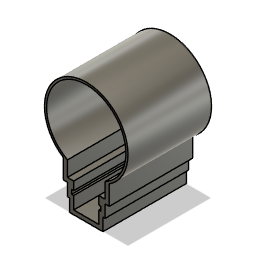
神秘PCB扣具 (Autodesk Fusion 360 design; units mm, degrees)
Autodesk Fusion 360 part; units mm, degrees
sketch "草图1" plane through (0, 0, 0) normal (0, 1, 0) x (1, 0, 0)
  circle A0 centre (0, 0) radius 10
  dimension "d1" = 20
  constraint coincident A0.centre origin
  measures "d1" diameter of A0
extrude "拉伸1" add sketch "草图1" along normal blind 20 makes body 1
sketch "草图2" plane through (0, 20, 0) normal (0, 1, 0) x (-1, 0, 0)
  circle A0 centre (0, 0) radius 10
  circle A1 centre (0, 0) radius 9.5
  dimension "d4" = 19
  constraint concentric A0 A1
  measures "d4" diameter of A1
extrude "拉伸2" cut sketch "草图2" against normal blind 20 contours A1 bodies 1
sketch "草图3" plane through (0, 20, 0) normal (0, 1, 0) x (-1, 0, 0)
  circle A0 centre (0, 0) radius 9.5
  circle A1 centre (0, 0) radius 10
  line L0 (4, 9) -> (-4, 9)
  line L1 (-4, 9) -> (-4, 19)
  line L2 (-4, 19) -> (4, 19)
  line L3 (4, 19) -> (4, 9)
  line L4 (3, 10) -> (-3, 10)
  line L5 (-3, 10) -> (-3, 18)
  line L6 (-3, 18) -> (3, 18)
  line L7 (3, 18) -> (3, 10)
  line L8 (3, 14) -> (3.5, 14)
  line L9 (3.5, 14) -> (3.5, 15)
  line L10 (3.5, 15) -> (3, 15)
  line L11 (3, 15) -> (3, 14)
  line L12 (-3, 14) -> (-3.5, 14)
  line L13 (-3.5, 14) -> (-3.5, 15)
  line L14 (-3.5, 15) -> (-3, 15)
  line L15 (-3, 15) -> (-3, 14)
  dimension "d7" = 8
  dimension "d8" = 4
  dimension "d9" = 9
  dimension "d10" = 10
  dimension "d11" = 1
  dimension "d12" = 1
  dimension "d13" = 1
  dimension "d14" = 1
  dimension "d15" = 0.5
  dimension "d16" = 1
  dimension "d17" = 0.5
  dimension "d18" = 1
  constraint horizontal L0
  constraint vertical L1
  constraint horizontal L2
  constraint vertical L3
  constraint horizontal L4
  constraint vertical L5
  constraint horizontal L6
  constraint vertical L7
  constraint horizontal L8
  constraint vertical L9
  constraint horizontal L10
  constraint vertical L11
  constraint midpoint L7 L8.start
  constraint horizontal L12
  constraint vertical L13
  constraint horizontal L14
  constraint vertical L15
  constraint midpoint L5 L12.start
  measures "d7" distance of L0.start L0.end
  measures "d8" distance of A0.centre L3
  measures "d9" distance of A0.centre L0
  measures "d10" distance of L0 L2
  measures "d11" distance of L0 L4
  measures "d12" distance of L2 L6
  measures "d13" distance of L1 L5
  measures "d14" distance of L3 L7
  measures "d15" distance of L9.end L10.end
  measures "d16" distance of L8 L10
  measures "d17" distance of L13.end L14.end
  measures "d18" distance of L12 L14
extrude "拉伸3" add sketch "草图3" against normal blind 20 contours A1 L1 L2 L3 bodies 1
sketch "草图4" plane through (0, 20, 0) normal (0, 1, 0) x (-1, 0, 0)
  line L0 (-3, 18) -> (3, 18)
  line L1 (3, 14) -> (3, 10)
  line L2 (3, 10) -> (-3, 10)
  line L3 (-3, 10) -> (-3, 14)
  line L4 (4, 9.1652) -> (4, 19)
  line L5 (4, 19) -> (-4, 19)
  line L6 (-4, 19) -> (-4, 9.1652)
  arc A0 (-4, 9.1652) -> (4, 9.1652) centre (0, 0) ccw
  line L7 (3, 14) -> (-3, 14)
  line L8 (-3, 14) -> (-3, 7.5)
  line L9 (-3, 7.5) -> (3, 7.5)
  line L10 (3, 7.5) -> (3, 14)
  line L11 (-3, 14) -> (-3.5, 14)
  line L12 (-3.5, 14) -> (-3.5, 15)
  line L13 (-3.5, 15) -> (-3, 15)
  line L14 (-3, 15) -> (-3, 18)
  line L15 (3, 18) -> (3, 15)
  line L16 (3, 15) -> (3.5, 15)
  line L17 (3.5, 15) -> (3.5, 14)
  line L18 (3.5, 14) -> (3, 14)
  circle A1 centre (0, 0) radius 9.5
  constraint horizontal L7
  constraint vertical L8
  constraint horizontal L9
  constraint vertical L10
  constraint coincident L1.start L7.start
extrude "拉伸4" cut sketch "草图4" against normal blind 20 contours L8 L9 L10 A1 picked at (-0.1243, 1.8358) bodies 1
sketch "草图5" plane through (0, 20, 0) normal (0, 1, 0) x (-1, 0, 0)
  line L0 (3, 10) -> (-3, 10)
  line L1 (-3, 10) -> (-3, 14)
  line L2 (-3, 14) -> (-3.5, 14)
  line L3 (-3.5, 14) -> (-3.5, 15)
  line L4 (-3.5, 15) -> (-3, 15)
  line L5 (-3, 15) -> (-3, 18)
  line L6 (-3, 18) -> (3, 18)
  line L7 (3, 18) -> (3, 15)
  line L8 (3, 15) -> (3.5, 15)
  line L9 (3.5, 15) -> (3.5, 14)
  line L10 (3.5, 14) -> (3, 14)
  line L11 (3, 14) -> (3, 10)
  circle A0 centre (0, 0) radius 9.5
  line L12 (4, 9.1652) -> (4, 19)
  line L13 (4, 19) -> (-4, 19)
  line L14 (-4, 19) -> (-4, 9.1652)
  arc A1 (-4, 9.1652) -> (4, 9.1652) centre (0, 0) ccw
  line L15 (4, 10) -> (-4, 10)
  line L16 (-4, 10) -> (-4, 13)
  line L17 (-4, 13) -> (4, 13)
  line L18 (4, 13) -> (4, 10)
  constraint horizontal L15
  constraint vertical L16
  constraint horizontal L17
  constraint vertical L18
  constraint coincident L14 L16.end
  constraint coincident L12 L15.start
extrude "拉伸5" cut sketch "草图5" against normal blind 20 contours L0 L1 L11 L15 L17 | L11 L12 L15 L17 L18 | L1 L14 L15 L16 L17 bodies 1 makes body 2 at (1.3333, 13.3333, 19)
sketch "草图6" plane through (0, 20, 0) normal (0, 1, 0) x (-1, 0, 0)
  circle A0 centre (0, 0) radius 9.5
  line L0 (4, 10) -> (-4, 10)
  line L1 (-4, 10) -> (-4, 9.1652)
  arc A1 (-4, 9.1652) -> (4, 9.1652) centre (0, 0) ccw
  line L2 (4, 9.1652) -> (4, 10)
  line L3 (5.5, 8) -> (-5.5, 8)
  line L4 (-5.5, 8) -> (-5.5, 13)
  line L5 (-5.5, 13) -> (5.5, 13)
  line L6 (5.5, 13) -> (5.5, 8)
  dimension "d25" = 5
  constraint horizontal L3
  constraint vertical L4
  constraint horizontal L5
  constraint vertical L6
  measures "d25" distance of L3.start L5.end
extrude "拉伸6" add sketch "草图6" against normal blind 20 contours L0 L1 A1 L2 L4 L5 L6 bodies 1 2
sketch "草图7" plane through (0, 20, 0) normal (0, 1, 0) x (-1, 0, 0)
  line L0 (-3, 13) -> (-3, 14)
  line L1 (-3, 14) -> (-3.5, 14)
  line L2 (-3.5, 14) -> (-3.5, 15)
  line L3 (-3.5, 15) -> (-3, 15)
  line L4 (-3, 15) -> (-3, 18)
  line L5 (-3, 18) -> (3, 18)
  line L6 (3, 18) -> (3, 15)
  line L7 (3, 15) -> (3.5, 15)
  line L8 (3.5, 15) -> (3.5, 14)
  line L9 (3.5, 14) -> (3, 14)
  line L10 (3, 14) -> (3, 13)
  line L11 (3, 13) -> (-3, 13)
  circle A0 centre (0, 0) radius 9.5
  line L12 (5.5, 8.3516) -> (5.5, 13)
  line L13 (5.5, 13) -> (4, 13)
  line L14 (4, 13) -> (4, 19)
  line L15 (4, 19) -> (-4, 19)
  line L16 (-4, 19) -> (-4, 13)
  line L17 (-4, 13) -> (-5.5, 13)
  line L18 (-5.5, 13) -> (-5.5, 8.3516)
  arc A1 (-5.5, 8.3516) -> (5.5, 8.3516) centre (0, 0) ccw
  line L19 (4.5, 8.0706) -> (-4.5, 8.0706)
  line L20 (-4.5, 8.0706) -> (-4.5, 12)
  line L21 (-4.5, 12) -> (4.5, 12)
  line L22 (4.5, 12) -> (4.5, 8.0706)
  dimension "d28" = 1
  dimension "d29" = 1
  dimension "d30" = 1
  constraint horizontal L19
  constraint vertical L20
  constraint horizontal L21
  constraint vertical L22
  measures "d28" distance of L12 L22
  measures "d29" distance of L18 L20
  measures "d30" distance of L13 L21
extrude "拉伸7" cut sketch "草图7" against normal blind 20 contours A0 L20 L21 L22 bodies 1
sketch "草图8" plane through (0, 20, 0) normal (0, 1, 0) x (-1, 0, 0)
  line L0 (4.5, 12) -> (4.5, 8.3666)
  arc A0 (-4.5, 8.3666) -> (4.5, 8.3666) centre (0, 0) ccw
  line L1 (-4.5, 8.3666) -> (-4.5, 12)
  line L2 (-4.5, 12) -> (4.5, 12)
  line L3 (-3, 13) -> (-3, 14)
  line L4 (-3, 14) -> (-3.5, 14)
  line L5 (-3.5, 14) -> (-3.5, 15)
  line L6 (-3.5, 15) -> (-3, 15)
  line L7 (-3, 15) -> (-3, 18)
  line L8 (-3, 18) -> (3, 18)
  line L9 (3, 18) -> (3, 15)
  line L10 (3, 15) -> (3.5, 15)
  line L11 (3.5, 15) -> (3.5, 14)
  line L12 (3.5, 14) -> (3, 14)
  line L13 (3, 14) -> (3, 13)
  line L14 (3, 13) -> (-3, 13)
  line L15 (5.5, 8.3516) -> (5.5, 13)
  line L16 (5.5, 13) -> (4, 13)
  line L17 (4, 13) -> (4, 19)
  line L18 (4, 19) -> (-4, 19)
  line L19 (-4, 19) -> (-4, 13)
  line L20 (-4, 13) -> (-5.5, 13)
  line L21 (-5.5, 13) -> (-5.5, 8.3516)
  arc A1 (-5.5, 8.3516) -> (5.5, 8.3516) centre (0, 0) ccw
  line L22 (3, 12) -> (-3, 12)
  line L23 (-3, 12) -> (-3, 13)
  line L24 (-3, 13) -> (3, 13)
  line L25 (3, 13) -> (3, 12)
  constraint horizontal L22
  constraint vertical L23
  constraint horizontal L24
  constraint vertical L25
  constraint coincident L3.start L14.end
  constraint coincident L2 L22.start
extrude "拉伸8" cut sketch "草图8" against normal blind 20 contours L2 L14 L22 L23 L24 L25 bodies 1
sketch "草图9" plane through (0, 20, 0) normal (0, 1, 0) x (-1, 0, 0)
  line L0 (5.5, 8.3516) -> (5.5, 13)
  line L1 (5.5, 13) -> (4, 13)
  line L2 (4, 13) -> (4, 19)
  line L3 (4, 19) -> (-4, 19)
  line L4 (-4, 19) -> (-4, 13)
  line L5 (-4, 13) -> (-5.5, 13)
  line L6 (-5.5, 13) -> (-5.5, 8.3516)
  arc A0 (-5.5, 8.3516) -> (5.5, 8.3516) centre (0, 0) ccw
  line L7 (3, 14) -> (3, 12)
  line L8 (3, 12) -> (4.5, 12)
  line L9 (4.5, 12) -> (4.5, 8.3666)
  arc A1 (-4.5, 8.3666) -> (4.5, 8.3666) centre (0, 0) ccw
  line L10 (-4.5, 8.3666) -> (-4.5, 12)
  line L11 (-4.5, 12) -> (-3, 12)
  line L12 (-3, 12) -> (-3, 14)
  line L13 (-3, 14) -> (-3.5, 14)
  line L14 (-3.5, 14) -> (-3.5, 15)
  line L15 (-3.5, 15) -> (-3, 15)
  line L16 (-3, 15) -> (-3, 18)
  line L17 (-3, 18) -> (3, 18)
  line L18 (3, 18) -> (3, 15)
  line L19 (3, 15) -> (3.5, 15)
  line L20 (3.5, 15) -> (3.5, 14)
  line L21 (3.5, 14) -> (3, 14)
  line L22 (4.5, 13) -> (-4.5, 13)
  line L23 (-4.5, 13) -> (-4.5, 16)
  line L24 (-4.5, 16) -> (4.5, 16)
  line L25 (4.5, 16) -> (4.5, 13)
  dimension "d35" = 2
  constraint horizontal L22
  constraint vertical L23
  constraint horizontal L24
  constraint vertical L25
  constraint coincident L1 L22.start
  measures "d35" distance of L17 L24
extrude "拉伸9" add sketch "草图9" against normal blind 20 contours L1 L2 L22 L24 L25 | L4 L5 L22 L23 L24 bodies 1
move_body "移动1" bodies 1 to x (1, 0, 0) y (0, 0, 1) z (0, -1, 0) at (0, 25, 5)
